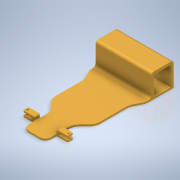
# Autodesk Inventor part: base_plate
Saved by Autodesk Inventor 2020 (Build 240168000, 168)
## iProperties
Created: 2020-03-15
Part Number: base_plate
Material: Acrylic, Clear
Document SubType Name: Modeling
Designer: 0x6f736f646f
Density: 1.19 g/cm^3
Appearance: Brass - Satin
Author: 0x6f736f646f
Autodesk Inventor part; units mm, degrees
ref_plane "XZ Plane" through (0, 0, 0) normal (0, 1, 0) x (-1, 0, 0)
sketch "Sketch1" plane through (0, 0, 0) normal (0, 1, 0) x (-1, 0, 0)
  line L0 (0, -154.7214) -> (0, -200)
  line L1 (0, -200) -> (-100, -200)
  line L2 (-100, -200) -> (-100, -154.7214)
  line L3 (-60, 0) -> (-40, 0)
  line L4 (-2.1115, -145.7771) -> (-7.8885, -134.2229)
  line L5 (-10, -125.2786) -> (-10, -78.2843)
  line L6 (-15.8579, -64.1421) -> (-24.1421, -55.8579)
  line L7 (-30, -41.7157) -> (-30, -10)
  line L8 (-70, -10) -> (-70, -41.7157)
  line L9 (-75.8579, -55.8579) -> (-84.1421, -64.1421)
  line L10 (-90, -78.2843) -> (-90, -125.2786)
  line L11 (-92.1115, -134.2229) -> (-97.8885, -145.7771)
  arc A0 (-30, -41.7157) -> (-24.1421, -55.8579) centre (-10, -41.7157) ccw
  arc A1 (-75.8579, -55.8579) -> (-70, -41.7157) centre (-90, -41.7157) ccw
  arc A2 (-84.1421, -64.1421) -> (-90, -78.2843) centre (-70, -78.2843) ccw
  arc A3 (-10, -78.2843) -> (-15.8579, -64.1421) centre (-30, -78.2843) ccw
  arc A4 (-10, -125.2786) -> (-7.8885, -134.2229) centre (10, -125.2786) ccw
  arc A5 (-92.1115, -134.2229) -> (-90, -125.2786) centre (-110, -125.2786) ccw
  arc A6 (-97.8885, -145.7771) -> (-100, -154.7214) centre (-80, -154.7214) ccw
  arc A7 (0, -154.7214) -> (-2.1115, -145.7771) centre (-20, -154.7214) ccw
  arc A8 (-30, -10) -> (-40, 0) centre (-40, -10) ccw
  arc A9 (-60, 0) -> (-70, -10) centre (-60, -10) ccw
  point P0 (0, 0)
  point P1 (-100, 0)
  point P2 (0, -150)
  point P3 (-10, -130)
  point P4 (-10, -70)
  point P5 (-30, -50)
  point P6 (-30, 0)
  point P7 (-70, 0)
  point P8 (-70, -50)
  point P9 (-90, -70)
  point P10 (-90, -130)
  point P11 (-100, -150)
  point P12 (0, 0)
  dimension "d23" = 50
  dimension "d24" = 60
  dimension "d25" = 60
  dimension "d26" = 50
  dimension "d27" = 50
  dimension "d28" = 50
  dimension "d29" = 20
  dimension "d30" = 20
  dimension "d31" = 40
  dimension "d32" = 100
  dimension "d34" = 10
  dimension "d35" = 10
  dimension "d36" = 20
  dimension "d37" = 200
  dimension "d38" = 20
  dimension "d39" = 10
  constraints: 24 end point, 24 point on line, 20 point on circle, 20 tangent, 10 centre point, 8 equal radius, 4 perpendicular, 3 vertical, 1 coincident, 1 parallel
  measures "d23" distance of point (-30, -50) point (-30, 0)
  measures "d24" distance of point (-10, -130) point (-10, -70)
  measures "d25" distance of point (-90, -70) point (-90, -130)
  measures "d26" distance of point (-70, 0) point (-70, -50)
  measures "d27" distance of L1.end point (-100, -150)
  measures "d28" distance of L0.end point (0, -150)
  measures "d29" vertical distance of point (-10, -130) point (0, -150)
  measures "d30" vertical distance of point (-100, -150) point (-90, -130)
  measures "d31" distance between parallel lines of L8 L7
  measures "d32" distance between parallel lines of L2 L0
  measures "d34" distance between parallel lines of L0 L5
  measures "d35" distance between parallel lines of L2 L10
  measures "d36" distance between parallel lines of L5 L7
  measures "d37" distance between parallel lines of L1 L3
  measures "d38" radius of A0
  measures "d39" radius of A8
extrude "Extrusion2" add sketch "Sketch1" against normal blind 3
ref_plane "Work Plane1" through (0, 0, -25) normal (0, 0, 1) x (1, 0, 0)
sketch "Sketch4" plane through (0, 0, -25) normal (0, 0, 1) x (1, 0, 0)
  line L0 (70, -3) -> (70, 5)
  line L1 (72, 7) -> (90, 7)
  line L2 (90, 7) -> (90, 4.5)
  line L3 (90, 4.5) -> (77, 4.5)
  line L4 (75, 2.5) -> (75, 1.5)
  line L5 (77, -0.5) -> (90, -0.5)
  line L6 (90, -0.5) -> (90, -3)
  line L7 (90, -3) -> (70, -3)
  arc A0 (72, 7) -> (70, 5) centre (72, 5) ccw
  arc A1 (77, 4.5) -> (75, 2.5) centre (77, 2.5) ccw
  arc A2 (75, 1.5) -> (77, -0.5) centre (77, 1.5) ccw
  line L8 (60, -3) -> (70, -3) projected
  line L9 (70, 0) -> (70, -3) projected
  point P0 (0, 0)
  dimension "d66" = 5
  dimension "d67" = 2.5
  dimension "d68" = 2.5
  dimension "d69" = 20
  dimension "d70" = 15
  dimension "d71" = 2
  constraints: 16 end point, 6 point on circle, 6 tangent, 4 point on line, 3 centre point, 3 perpendicular, 2 equal radius, 2 horizontal, 1 parallel, 1 vertical
  measures "d66" distance between parallel lines of L5 L3
  measures "d67" distance between parallel lines of L3 L1
  measures "d68" distance between parallel lines of L7 L5
  measures "d69" distance between parallel lines of L2 L0
  measures "d70" distance between parallel lines of L2 L4
  measures "d71" radius of A0
extrude "Extrusion3" add sketch "Sketch4" along normal mid plane 10
fillet "Fillet1" radius 2 1 edges at (70, 0, -25)
fillet "Fillet2" radius 2 1 edges at (70, -1.5, -20)
fillet "Fillet3" radius 0.5 2 edges at (71, 0, -20) (69, 0, -20)
fillet "Fillet4" radius 1.26 1 edges at (70, -1.5, -30)
fillet "Fillet5" radius 0.5 2 edges at (70.63, 0, -30) (69, 0, -30)
sketch "Sketch5" plane through (72, 7, -20) normal (0, 1, 0) x (1, 0, 0)
  line L0 (18, 10) -> (18, 0) projected
  line L1 (0, 10) -> (18, 10) projected
  point P0 (-72, -20)
  point P1 (15, 5)
  dimension "d86" = 3
  dimension "d87" = 5
  measures "d86" distance from line of L0 point (15, 5)
  measures "d87" distance from line of point (15, 5) L1
hole "Hole1" at (87, 7, -25) direction (0, -1, 0) diameter 3 end through all both
ref_plane "Work Plane2" through (50, 0, 0) normal (1, 0, 0) x (0, 1, 0)
mirror "Mirror1" about plane through (50, 0, 0) normal (1, 0, 0) of "Extrusion3", "Hole1"
fillet "Fillet6" radius 2 1 edges at (30, 0, -25)
fillet "Fillet7" radius 2.12 1 edges at (30, -1.5, -20)
fillet "Fillet8" radius 1 2 edges at (28.94, 0, -20) (31, 0, -20)
fillet "Fillet9" radius 2.46 1 edges at (30, -1.5, -30)
fillet "Fillet10" radius 1 2 edges at (28.77, 0, -30) (31, 0, -30)
fillet "Fillet11" radius 2 8 edges at (10, 5.75, -30) (10, -1.75, -30) (10, -1.75, -20) (10, 5.75, -20) (90, 5.75, -20) (90, -1.75, -20) (90, -1.75, -30) (90, 5.75, -30)
sketch "Sketch6" plane through (50, 0, 0) normal (1, 0, 0) x (0, 1, 0)
  line L0 (40, -160) -> (0, -160)
  line L1 (0, -160) -> (0, -200)
  line L2 (0, -200) -> (40, -200)
  line L3 (40, -200) -> (40, -160)
  line L4 (35, -165) -> (5, -165)
  line L5 (5, -195) -> (35, -195)
  line L6 (35, -195) -> (35, -165)
  line L7 (5, -165) -> (0, -165)
  line L8 (5, -195) -> (0, -195)
  line L9 (0, -154.7214) -> (0, -200) projected
  point P0 (0, 0)
  dimension "d95" = 40
  dimension "d96" = 40
  dimension "d97" = 5
  dimension "d98" = 5
  dimension "d100" = 5
  constraints: 18 end point, 4 parallel, 2 horizontal, 2 perpendicular, 2 point on line, 1 coincident
  measures "d95" distance of L2.end L0.start
  measures "d96" distance between parallel lines of L1 L3
  measures "d97" distance between parallel lines of L6 L3
  measures "d98" distance between parallel lines of L0 L4
  measures "d100" distance between parallel lines of L2 L5
extrude "Extrusion4" add sketch "Sketch6" along normal mid plane 100 contours L3 L2 L1 L8 L5 L6 L4 L7 L0
fillet "Fillet12" radius 5 1 edges at (50, 40, -200)
fillet "Fillet13" radius 5 1 edges at (50, 40, -160)
fillet "Fillet14" radius 5 1 edges at (50, 0, -160)
body "Solid2"
